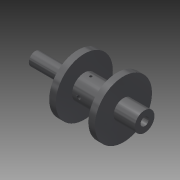
# Autodesk Inventor part: 13_0204_055
Saved by Autodesk Inventor 2012 SP1 (Build 160190100, 190)
## iProperties
Created: 2013-04-15
Part Number: 13_0204_055
Material: Default
Document SubType Name: Modeling
Designer: vogel
Density: 1 g/cm^3
Author: vogel
Autodesk Inventor part; units mm, degrees
note: some values were not read from the file. Chosen so that the rebuilt part matches the saved one: direction of "Bohrung4".
sketch "Skizze1" plane through (0, 0, 0) normal (0, 0, 1) x (1, 0, 0)
  line L0 (-53.4, 0) -> (40.4, 0) projected
  line L1 (0, -3.5) -> (0, 21) projected
  line L2 (-10, 7.5) -> (10, 7.5)
  line L3 (10, 7.5) -> (10, 17.5)
  line L4 (10, 17.5) -> (14, 17.5)
  line L5 (14, 17.5) -> (14, 6)
  line L6 (14, 6) -> (27, 6)
  line L7 (27, 6) -> (27, 0)
  line L8 (-10, 7.5) -> (-10, 17.5)
  line L9 (-10, 17.5) -> (-14, 17.5)
  line L10 (-14, 17.5) -> (-14, 4)
  line L11 (-14, 4) -> (-40, 4)
  line L12 (-40, 4) -> (-40, 0)
  line L13 (-40, 0) -> (27, 0)
  point P0 (0, 0)
  dimension "d0" = 20
  dimension "d1" = 15
  dimension "d2" = 28
  dimension "d3" = 10
  dimension "d4" = 8
  dimension "d5" = 40
  dimension "d6" = 12
  dimension "d7" = 27
  constraints: 24 end point, 6 parallel, 5 perpendicular, 2 collinear, 2 point on line, 2 other
  measures "d0" distance between parallel lines of L3 L8
  measures "d1" diameter of L2 L13
  measures "d2" distance between parallel lines of L5 L10
  measures "d3" distance between parallel lines of L2 L9
  measures "d4" diameter of L11 L13
  measures "d5" distance between parallel lines of L12 L1
  measures "d6" diameter of L6 L13
  measures "d7" distance between parallel lines of L1 L7
revolve "Umdrehung1" add sketch "Skizze1" angle 360 about axis through (-40, 0, 0) along (1, 0, 0)
ref_plane "Arbeitsebene1" through (0, 0, 7.5) normal (0, 0, 1) x (1, 0, 0)
ref_plane "Arbeitsebene2" through (0, -7.5, 0) normal (0, 1, 0) x (-1, 0, 0)
sketch "Skizze2" plane through (0, 0, 7.5) normal (0, 0, 1) x (1, 0, 0)
  line L0 (-53.4, 0) -> (40.4, 0) projected
  line L1 (0, -24.5) -> (0, 24.5) projected
  point P0 (0, 0)
  point P1 (-6, 0)
  dimension "d9" = 6
  constraints: 1 point on line
  measures "d9" distance from line of point (-6, 0) L1
hole "Bohrung1" at (-6, 0, 7.5) direction (0, 0, -1) diameter 1.5 end through all
sketch "Skizze3" plane through (0, -7.5, 0) normal (0, 1, 0) x (-1, 0, 0)
  line L0 (53.4, 0) -> (-40.4, 0) projected
  line L1 (0, -24.5) -> (0, 24.5) projected
  point P0 (0, 0)
  point P1 (6, 0)
  dimension "d17" = 6
  constraints: 1 point on line
  measures "d17" distance from line of point (6, 0) L1
hole "Bohrung2" at (-6, -7.5, 0) direction (0, 1, 0) diameter 2.459 end through all thread size "M3x0.5" class "6H" standard "ISO Metric profile"
hole "Bohrung3" at (27, 0, 0) direction (-1, 0, 0) diameter 5 depth 25 tip angle 118
ref_plane "Arbeitsebene3" through (20.5, 6, 0) normal (0, 1, 0) x (-1, 0, 0)
sketch "Skizze6" plane through (20.5, 6, 0) normal (0, 1, 0) x (-1, 0, 0)
  line L0 (-6.5, 6) -> (-6.5, -6) projected
  line L1 (73.9, 0) -> (-19.9, 0) projected
  line L2 (20.5, -24.5) -> (20.5, 24.5) projected
  point P0 (20.5, 0)
  point P1 (-0.5, 0)
  dimension "d36" = 6
  constraints: 1 point on line
  measures "d36" distance from line of L0 point (-0.5, 0)
hole "Bohrung4" at (21, 6, 0) direction (0, -1, 0) diameter 2.459 end up to surface thread size "M3x0.5" class "6H" standard "ISO Metric profile"
